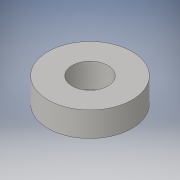
# Autodesk Inventor part: Connector-qty1
Saved by Autodesk Inventor 2016 (Build 200138000, 138)
## iProperties
Created: 2016-05-25
Part Number: Connector-qty1
Material: Generic
Document SubType Name: Modeling
Designer: jregalado
Density: 1 g/cm^3
Appearance: Default
Author: jregalado
Autodesk Inventor part; units mm, degrees
ref_plane "YZ Plane" through (0, 0, 0) normal (1, 0, 0) x (0, 1, 0)
ref_plane "XZ Plane" through (0, 0, 0) normal (0, 1, 0) x (-1, 0, 0)
ref_plane "XY Plane" through (0, 0, 0) normal (0, 0, 1) x (1, 0, 0)
sketch "Sketch1" plane through (0, 0, 0) normal (0, 1, 0) x (-1, 0, 0)
  circle A0 centre (0, -12.2555) radius 1.8415
  circle A1 centre (0, -12.2555) radius 4.318
  point P0 (0, 0)
  point P1 (2.54, -8.7636)
  dimension "d7" = 8.636
  constraints: 1 centre point, 1 coincident, 3 other
extrude "Extrusion2" add sketch "Sketch1" along normal blind 2.54
body "Solid2"
